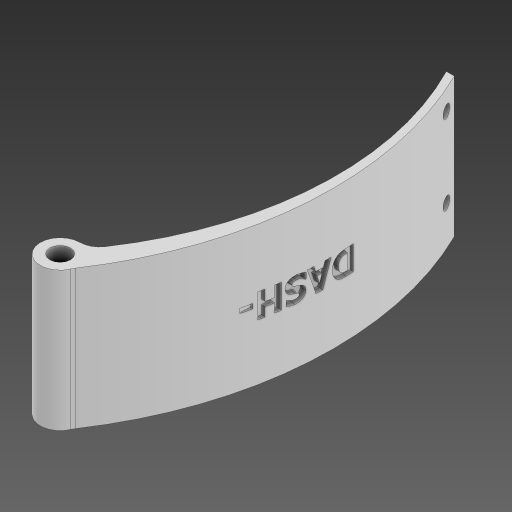
# Autodesk Inventor part: protect
Saved by Autodesk Inventor 2023 (Build 270158000, 158)
## iProperties
Created: 2025-06-27
Part Number: protect
Material: Типовые
Document SubType Name: Modeling
Designer: daa
Density: 1 g/cm^3
Appearance: По умолчанию
Author: daa
Autodesk Inventor part; units mm, degrees
ref_plane "YZ Plane" through (0, 0, 0) normal (1, 0, 0) x (0, 1, 0)
ref_plane "XZ Plane" through (0, 0, 0) normal (0, 1, 0) x (-1, 0, 0)
ref_plane "XY Plane" through (0, 0, 0) normal (0, 0, 1) x (1, 0, 0)
sketch "Эскиз1" plane through (0, 0, 0) normal (0, 1, 0) x (-1, 0, 0)
  circle A0 centre (-56.0718, 132.2835) radius 2.6
  line L0 (-64.9084, 43.85) -> (-66.9084, 43.85)
  circle A1 centre (-56.0718, 132.2835) radius 5.0026
  arc A2 (-60.8228, 133.85) -> (-66.9084, 43.85) centre (13.8399, 83.5958) ccw
  arc A3 (-58.2432, 127.7768) -> (-64.9084, 43.85) centre (6.2398, 80.4278) ccw
  line L1 (-60.8228, 133.85) -> (-51.3208, 133.85)
  point P0 (-68.2724, 116.2724)
  dimension "d27" = 5.2
  dimension "d28" = 2
  dimension "d29" = 90
  dimension "d30" = 80
  dimension "d35" = 90
  dimension "d47" = 10.0052
  dimension "d48" = 1.5665
  constraints: 7 point on circle, 4 centre point, 4 end point, 2 coincident, 2 horizontal
  measures "d27" diameter of A0
  measures "d28" distance of L0.start L0.end
  measures "d29" radius of A2
  measures "d30" radius of A3
  measures "d35" vertical distance of L0.end L1.start
  measures "d47" diameter of A1
  measures "d48" distance from line of L1 A0.centre
extrude "Выдавливание1" add sketch "Эскиз1" along normal blind 35 contours A0 L1 A1 | A0 L1 A1 | A1 A3 L0 A2
sketch "Эскиз2" plane through (0, 0, 0) normal (1, 0, 0) x (0, 1, 0)
  circle A0 centre (30, 47.55) radius 1.5
  circle A1 centre (10, 47.55) radius 1.5
  line L0 (0, 43.85) -> (35, 43.85) projected
  line L1 (35, 127.7768) -> (35, 43.85) projected
  point P0 (0, 0)
  dimension "d36" = 3
  dimension "d37" = 3
  dimension "d38" = 3.7
  dimension "d39" = 3.7
  dimension "d40" = 5
  dimension "d41" = 20
  constraints: 2 centre point
  measures "d36" diameter of A0
  measures "d37" diameter of A1
  measures "d38" distance from line of L0 A1.centre
  measures "d39" distance from line of L0 A0.centre
  measures "d40" distance from line of L1 A0.centre
  measures "d41" distance of A0.centre A1.centre
extrude "Выдавливание2" cut sketch "Эскиз2" along normal blind 94.5
fillet "Сопряжение3" radius 5 1 edges at (58.2432, 17.5, 127.7768)
fillet "Сопряжение4" radius 5 1 edges at (60.8228, 17.5, 133.85)
ref_plane "РабПлоскость3" through (78.8834, 0, 44.6231) normal (0.9979225, 0, 0.0644264) x (0, 1, 0)
ref_plane "РабПлоскость2" through (66.9084, 0, 43.85) normal (0.9979225, 0, 0.0644264) x (0, 1, 0)
sketch "Эскиз4" plane through (78.8834, 0, 44.6231) normal (0.9979225, 0, 0.0644264) x (0, 1, 0)
  line L0 (14.0417, 33.2562) -> (14.0417, 55.6622) construction
  line L1 (14.0417, 55.6622) -> (14.5551, 55.6622) construction
  line L2 (14.5551, 55.6622) -> (14.5551, 33.2562) construction
  line L3 (14.5551, 33.2562) -> (14.0417, 33.2562) construction
  spline S0 degree 2 poles (17.2054, 39.3315) (18.0606, 39.3315) (19.4052, 38.585) (19.766, 38.0166) knots 0 0 0 1 2 2 2
  spline S1 degree 2 poles (19.766, 38.0166) (20.0725, 37.542) (20.2505, 36.4248) (20.2505, 35.797) knots 0 0 0 1 2 2 2
  line L4 (20.2505, 35.797) -> (20.2505, 33.8889)
  line L5 (20.2505, 33.8889) -> (14.1505, 33.8889)
  line L6 (14.1505, 33.8889) -> (14.1505, 35.7772)
  spline S2 degree 2 poles (14.1505, 35.7772) (14.1505, 36.4199) (14.3136, 37.542) (14.63, 38.0363) knots 0 0 0 1 2 2 2
  spline S3 degree 2 poles (14.63, 38.0363) (15.0156, 38.6345) (16.3206, 39.3315) (17.2054, 39.3315) knots 0 0 0 1 2 2 2
  spline S4 degree 2 poles (17.1955, 37.7595) (16.5925, 37.7595) (15.7323, 37.3443) (15.4901, 36.9191) knots 0 0 0 1 2 2 2
  spline S5 degree 2 poles (15.4901, 36.9191) (15.322, 36.6077) (15.2874, 35.9255) (15.2874, 35.451) knots 0 0 0 1 2 2 2
  line L7 (15.2874, 35.451) -> (15.2874, 35.4213)
  line L8 (15.2874, 35.4213) -> (19.1086, 35.4213)
  line L9 (19.1086, 35.4213) -> (19.1086, 35.451)
  spline S6 degree 2 poles (19.1086, 35.451) (19.1086, 35.9651) (19.074, 36.672) (18.8713, 36.9933) knots 0 0 0 1 2 2 2
  spline S7 degree 2 poles (18.8713, 36.9933) (18.634, 37.369) (17.7986, 37.7595) (17.1955, 37.7595) knots 0 0 0 1 2 2 2
  line L10 (20.2505, 39.5836) -> (14.1505, 41.6449)
  line L11 (14.1505, 41.6449) -> (14.1505, 43.3157)
  line L12 (14.1505, 43.3157) -> (20.2505, 45.3771)
  line L13 (20.2505, 45.3771) -> (20.2505, 43.8002)
  line L14 (20.2505, 43.8002) -> (19.0048, 43.4196)
  line L15 (19.0048, 43.4196) -> (19.0048, 41.5016)
  line L16 (19.0048, 41.5016) -> (20.2505, 41.116)
  line L17 (20.2505, 41.116) -> (20.2505, 39.5836)
  line L18 (17.8975, 43.0834) -> (15.8806, 42.4606)
  line L19 (15.8806, 42.4606) -> (17.8975, 41.8328)
  line L20 (17.8975, 41.8328) -> (17.8975, 43.0834)
  spline S8 degree 2 poles (20.3592, 47.8685) (20.3592, 47.1666) (20.0874, 46.1087) (19.8896, 45.6539) knots 0 0 0 1 2 2 2
  line L21 (19.8896, 45.6539) -> (18.4363, 45.6539)
  line L22 (18.4363, 45.6539) -> (18.4363, 45.7923)
  spline S9 degree 2 poles (18.4363, 45.7923) (18.8268, 46.252) (19.247, 47.3544) (19.247, 47.8734) knots 0 0 0 1 2 2 2
  spline S10 degree 2 poles (19.247, 47.8734) (19.247, 48.0069) (19.1877, 48.437) (19.1284, 48.5655) knots 0 0 0 1 2 2 2
  spline S11 degree 2 poles (19.1284, 48.5655) (19.0592, 48.7237) (18.807, 48.9461) (18.6044, 48.9461) knots 0 0 0 1 2 2 2
  spline S12 degree 2 poles (18.6044, 48.9461) (18.372, 48.9461) (18.0853, 48.5853) (18.0211, 48.3381) knots 0 0 0 1 2 2 2
  spline S13 degree 2 poles (18.0211, 48.3381) (17.937, 48.0267) (17.7937, 47.3198) (17.6849, 47.0084) knots 0 0 0 1 2 2 2
  spline S14 degree 2 poles (17.6849, 47.0084) (17.4378, 46.3015) (16.5925, 45.6885) (15.9597, 45.6885) knots 0 0 0 1 2 2 2
  spline S15 degree 2 poles (15.9597, 45.6885) (15.1045, 45.6885) (14.0417, 47.1369) (14.0417, 48.2244) knots 0 0 0 1 2 2 2
  spline S16 degree 2 poles (14.0417, 48.2244) (14.0417, 48.7682) (14.2642, 49.8458) (14.452, 50.2709) knots 0 0 0 1 2 2 2
  line L23 (14.452, 50.2709) -> (15.846, 50.2709)
  line L24 (15.846, 50.2709) -> (15.846, 50.1375)
  spline S17 degree 2 poles (15.846, 50.1375) (15.5544, 49.7964) (15.154, 48.8176) (15.154, 48.3035) knots 0 0 0 1 2 2 2
  spline S18 degree 2 poles (15.154, 48.3035) (15.154, 48.1008) (15.2133, 47.7845) (15.2924, 47.6065) knots 0 0 0 1 2 2 2
  spline S19 degree 2 poles (15.2924, 47.6065) (15.3566, 47.4631) (15.6137, 47.2555) (15.7719, 47.2555) knots 0 0 0 1 2 2 2
  spline S20 degree 2 poles (15.7719, 47.2555) (16.0092, 47.2555) (16.281, 47.5867) (16.3898, 48.0613) knots 0 0 0 1 2 2 2
  spline S21 degree 2 poles (16.3898, 48.0613) (16.459, 48.3678) (16.5925, 48.9362) (16.7062, 49.2625) knots 0 0 0 1 2 2 2
  spline S22 degree 2 poles (16.7062, 49.2625) (16.9385, 49.8952) (17.7096, 50.5131) (18.3424, 50.5131) knots 0 0 0 1 2 2 2
  spline S23 degree 2 poles (18.3424, 50.5131) (19.2519, 50.5131) (20.3592, 49.0845) (20.3592, 47.8685) knots 0 0 0 1 2 2 2
  line L25 (20.2505, 56.4451) -> (20.2505, 54.9127)
  line L26 (20.2505, 54.9127) -> (17.5465, 54.9127)
  line L27 (17.5465, 54.9127) -> (17.5465, 52.8315)
  line L28 (17.5465, 52.8315) -> (20.2505, 52.8315)
  line L29 (20.2505, 52.8315) -> (20.2505, 51.2991)
  line L30 (20.2505, 51.2991) -> (14.1505, 51.2991)
  line L31 (14.1505, 51.2991) -> (14.1505, 52.8315)
  line L32 (14.1505, 52.8315) -> (16.3848, 52.8315)
  line L33 (16.3848, 52.8315) -> (16.3848, 54.9127)
  line L34 (16.3848, 54.9127) -> (14.1505, 54.9127)
  line L35 (14.1505, 54.9127) -> (14.1505, 56.4451)
  line L36 (14.1505, 56.4451) -> (20.2505, 56.4451)
  line L37 (18.1249, 60.2415) -> (18.1249, 57.5277)
  line L38 (18.1249, 57.5277) -> (16.9879, 57.5277)
  line L39 (16.9879, 57.5277) -> (16.9879, 60.2415)
  line L40 (16.9879, 60.2415) -> (18.1249, 60.2415)
  point P0 (0, -39.4483)
  constraints: 2 other
extrude "Выдавливание3" cut sketch "Эскиз4" against normal blind 1.5
